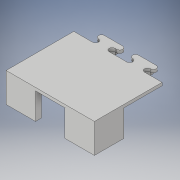
# Autodesk Inventor part: base auxiliar 1
Saved by Autodesk Inventor 2019 (Build 230136000, 136)
## iProperties
Created: 2018-08-28
Part Number: base auxiliar 1
Material: Genérico
Document SubType Name: Modeling
Designer: Albert Garangou Culebras
Density: 1 g/cm^3
Appearance: Valor por defecto
Author: Albert Garangou Culebras
Autodesk Inventor part; units mm, degrees
ref_plane "YZ Plane" through (0, 0, 0) normal (1, 0, 0) x (0, 1, 0)
ref_plane "XZ Plane" through (0, 0, 0) normal (0, 1, 0) x (-1, 0, 0)
ref_plane "XY Plane" through (0, 0, 0) normal (0, 0, 1) x (1, 0, 0)
sketch "puzzle" plane through (0, 0, 0) normal (0, 1, 0) x (-1, 0, 0)
  line L0 (0, 0) -> (-150, 0)
  line L1 (0, -115) -> (-15, -115)
  line L2 (-135, -115) -> (-125, -115)
  line L3 (-135, -115) -> (-150, -115)
  line L4 (-75, -115) -> (-65, -115)
  line L5 (-75, -115) -> (-85.0002, -115)
  line L6 (-105, -135) -> (-94.9796, -135)
  line L7 (-94.9796, -135) -> (-115, -135)
  line L8 (-65, -115) -> (-60, -115)
  line L9 (-60, -125) -> (-63, -125)
  arc A0 (-60, -125) -> (-60, -115) centre (-60, -120) ccw
  arc A1 (-63, -125) -> (-63, -135) centre (-63, -130) ccw
  line L10 (-85.0002, -115) -> (-90.0002, -115)
  line L11 (-94.9796, -135) -> (-89.9796, -135)
  arc A2 (-90.0002, -115) -> (-90, -125) centre (-90.0002, -120) ccw
  arc A3 (-89.9796, -135) -> (-90, -125) centre (-89.9796, -130) ccw
  line L12 (-115, -135) -> (-120, -135)
  line L13 (-125, -115) -> (-120, -115)
  arc A4 (-120, -125) -> (-120, -115) centre (-120, -120) ccw
  arc A5 (-120, -125) -> (-120, -135) centre (-120, -130) ccw
  line L14 (0, -115) -> (-30, -115)
  line L15 (-63, -135) -> (-32.98, -135)
  line L16 (-32.98, -135) -> (-32, -135)
  line L17 (-30, -115) -> (-32, -115)
  arc A6 (-32, -115) -> (-32, -125) centre (-32, -120) ccw
  arc A7 (-32, -135) -> (-32, -125) centre (-32, -130) ccw
  line L18 (-150, -115) -> (-150, 0)
  line L19 (0, -115) -> (0, 0)
  dimension "d22" = 5
  dimension "d23" = 5
  dimension "d24" = 5
  dimension "d25" = 5
  dimension "d26" = 5
  constraints: 40 end point, 16 point on circle, 15 horizontal, 10 tangent, 8 centre point, 2 vertical, 1 point on line
  measures "d22" distance of L4.end L8.end
  measures "d23" distance of L5.end L10.end
  measures "d24" distance of L6.end L11.end
  measures "d25" distance of L7.end L12.end
  measures "d26" distance of L2.end L13.end
extrude "Extrusión1" add sketch "puzzle" along normal blind 5
sketch "peus" plane through (0, 0, 0) normal (0, -1, 0) x (1, 0, 0)
  line L0 (150, 0) -> (145, 0)
  line L1 (150, 0) -> (100, 0)
  line L2 (0, -115) -> (0, 0) projected
  line L3 (0, 0) -> (50, 0)
  line L4 (50, 0) -> (50, -10)
  line L5 (0, 0) -> (10, 0)
  line L6 (10, -50) -> (0, -50)
  line L7 (0, -50) -> (0, 0)
  line L8 (50, -10) -> (10, -10)
  line L9 (10, -10) -> (10, -50)
  line L10 (100, 0) -> (100, -10)
  line L11 (100, -10) -> (140, -10)
  line L12 (140, -10) -> (140, -50)
  line L13 (140, -50) -> (150, -50)
  line L14 (150, 0) -> (150, -115) projected
  line L15 (150, 0) -> (150, -50)
  line L16 (0, 0) -> (150, 0) projected
  line L17 (45, -62.5) -> (45, -72.5)
  line L18 (105, -72.5) -> (105, -62.5)
  line L19 (80, -97.5) -> (70, -97.5)
  line L20 (80, -37.5) -> (70, -37.5)
  line L21 (80, -62.5) -> (70, -62.5)
  line L22 (70, -62.5) -> (70, -72.5)
  line L23 (70, -72.5) -> (80, -72.5)
  line L24 (80, -62.5) -> (80, -72.5)
  line L25 (83, -62.5) -> (83, -59.5)
  line L26 (83, -59.5) -> (80, -59.5)
  line L27 (70, -59.5) -> (67, -59.5)
  line L28 (67, -59.5) -> (67, -62.5)
  line L29 (67, -72.5) -> (67, -75.5)
  line L30 (67, -75.5) -> (70, -75.5)
  line L31 (80, -75.5) -> (83, -75.5)
  line L32 (83, -75.5) -> (83, -72.5)
  line L33 (83, -72.5) -> (105, -72.5)
  line L34 (83, -62.5) -> (105, -62.5)
  line L35 (80, -59.5) -> (80, -37.5)
  line L36 (70, -59.5) -> (70, -37.5)
  line L37 (67, -62.5) -> (45, -62.5)
  line L38 (67, -72.5) -> (45, -72.5)
  line L39 (70, -75.5) -> (70, -97.5)
  line L40 (80, -75.5) -> (80, -97.5)
  line L41 (83, -72.5) -> (105, -72.5)
  dimension "d70" = 3
  constraints: 78 end point, 7 perpendicular, 6 vertical, 4 horizontal, 3 point on line, 1 collinear
  measures "d70" distance of L29.start L29.end
extrude "Extrusión3" add sketch "peus" along normal blind 45
sketch "Boceto4" plane through (0, 0, 0) normal (0, -1, 0) x (1, 0, 0)
  line L0 (55, -135) -> (37, -135)
  line L1 (120, -135) -> (89.9796, -135) projected
  line L2 (115, -135) -> (95, -135)
  line L3 (90.0002, -115) -> (60, -115) projected
  line L4 (75.0001, -115) -> (83.5001, -115)
  line L5 (83.5001, -115) -> (66.5001, -115)
  line L6 (83.5001, -110) -> (66.5001, -110)
  line L7 (83.5001, -110) -> (83.5001, -115)
  line L8 (66.5001, -110) -> (66.5001, -115)
  line L9 (55, -130) -> (37, -130)
  line L10 (55, -130) -> (55, -135)
  line L11 (37, -130) -> (37, -135)
  line L12 (115, -130) -> (95, -130)
  line L13 (95, -130) -> (95, -135)
  line L14 (115, -130) -> (115, -135)
  point P0 (0, 0)
  constraints: 26 end point, 6 vertical, 4 point on line, 1 collinear, 1 horizontal, 1 midpoint
extrude "Extrusión4" add sketch "Boceto4" along normal blind 10
sketch "Boceto5" plane through (55, 0, -135) normal (0, 0, -1) x (-1, 0, 0)
  circle A0 centre (9, -5) radius 1.6
  circle A1 centre (-50, -5) radius 1.6
  point P0 (55, 0)
  dimension "d81" = 3.2
  dimension "d82" = 3.2
  constraints: 2 centre point
  measures "d81" diameter of A0
  measures "d82" diameter of A1
extrude "Extrusión5" cut sketch "Boceto5" against normal blind 14.25
sketch "Boceto6" plane through (95, 0, -130) normal (0, 0, 1) x (1, 0, 0)
  circle A0 centre (-49, -5) radius 1.6 projected
  circle A1 centre (-49, -5) radius 3.05
  circle A2 centre (10, -5) radius 1.6 projected
  circle A3 centre (10, -5) radius 3.05
  point P0 (-95, 0)
  dimension "d85" = 6.1
  dimension "d86" = 6.1
  constraints: 2 centre point, 2 coincident
  measures "d85" diameter of A1
  measures "d86" diameter of A3
extrude "Extrusión6" cut sketch "Boceto6" against normal blind 2
sketch "Boceto7" plane through (66.5001, 0, -110) normal (0, 0, 1) x (1, 0, 0)
  line L0 (17, -10) -> (0, -10) projected
  line L1 (8.5, -10) -> (8.5, 0)
  line L2 (0, 0) -> (17, 0) projected
  circle A0 centre (8.5, -5) radius 3.05
  point P0 (-66.5001, 0)
  dimension "d89" = 6.1
  constraints: 3 midpoint, 2 end point, 1 centre point
  measures "d89" diameter of A0
extrude "Extrusión7" cut sketch "Boceto7" against normal blind 2
sketch "Boceto8" plane through (66.5001, 0, -110) normal (0, 0, 1) x (1, 0, 0)
  circle A0 centre (8.5, -5) radius 3.05 projected
  circle A1 centre (8.5, -5) radius 1.6
  point P0 (-66.5001, 0)
  dimension "d92" = 3.2
  constraints: 1 centre point, 1 coincident
  measures "d92" diameter of A1
extrude "Extrusión8" cut sketch "Boceto8" against normal blind 13 contours A1
